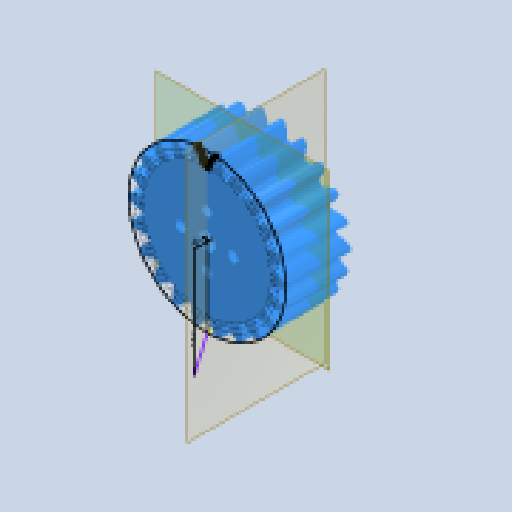
# Autodesk Inventor part: Шестерня
Saved by Autodesk Inventor 2024.2 (Build 282272000, 272)
## iProperties
Created: 2025-11-18
Part Number: Шестерня
Material: Generic
Document SubType Name: Modeling
Designer: katya_notebook
Density: 1 g/cm^3
Appearance: Голубой
Author: katya_notebook
Autodesk Inventor part; units mm, degrees
ref_plane "XZ Plane" through (0, 0, 0) normal (0, 1, 0) x (-1, 0, 0)
ref_plane "XY Plane" through (0, 0, 0) normal (0, 0, 1) x (1, 0, 0)
sketch "Sketch1" plane through (0, 0, 0) normal (0, 0, 1) x (1, 0, 0)
  spline S0 degree 3 poles (-2.783, 24.0561) (-2.7139, 23.9664) (-2.5759, 23.787) (-2.3787, 23.5105) (-2.1892, 23.2287) (-2.0087, 22.941) (-1.838, 22.6474) (-1.6779, 22.3479) (-1.5297, 22.0423) (-1.3949, 21.7305) (-1.2754, 21.4125) (-1.1922, 21.1419) (-1.1368, 20.9223) (-1.1074, 20.7551) (-1.0752, 20.5884) (-1.0286, 20.4249) (-0.9651, 20.2671) (-0.8815, 20.1188) (-0.7929, 20.0079) (-0.7126, 19.9278) (-0.645, 19.8764) (-0.5753, 19.8277) (-0.4987, 19.7907) (-0.4207, 19.7567) (-0.338, 19.7366) (-0.2548, 19.7191) (-0.1414, 19.715) (0, 19.7176) (0.1414, 19.715) (0.2548, 19.7191) (0.338, 19.7366) (0.4207, 19.7567) (0.4987, 19.7907) (0.5753, 19.8277) (0.645, 19.8764) (0.7126, 19.9278) (0.7929, 20.0079) (0.8815, 20.1188) (0.9651, 20.2671) (1.0286, 20.4249) (1.0752, 20.5884) (1.1074, 20.7551) (1.1368, 20.9223) (1.1922, 21.1419) (1.2754, 21.4125) (1.3949, 21.7305) (1.5297, 22.0423) (1.6779, 22.3479) (1.838, 22.6474) (2.0087, 22.941) (2.1892, 23.2287) (2.3787, 23.5105) (2.5759, 23.787) (2.7139, 23.9664) (2.783, 24.0561) knots 0 0 0 0 0.033955 0.067911 0.101866 0.135821 0.169776 0.203731 0.237685 0.271639 0.305591 0.339542 0.356519 0.373494 0.390468 0.407437 0.424408 0.441372 0.458331 0.46682 0.475308 0.483794 0.492283 0.500768 0.509256 0.517742 0.52623 0.543208 0.560186 0.568674 0.57716 0.585647 0.594133 0.602622 0.611107 0.619596 0.628084 0.645044 0.662008 0.678979 0.695948 0.712922 0.729897 0.746874 0.780824 0.814777 0.848731 0.882685 0.916639 0.950594 0.984549 1.018505 1.05246 1.086416 1.086416 1.086416 1.086416
  circle A0 centre (0, 0) radius 19.7166 construction
  circle A1 centre (0, 0) radius 20.6732 construction
  circle A2 centre (0, 0) radius 22 construction
  circle A3 centre (0, 0) radius 24.2166
  point P0 (-2.5775, 23.7858)
  point P1 (-2.38, 23.5096)
  point P2 (-2.1907, 23.2277)
  point P3 (-2.0103, 22.94)
  point P4 (-1.8398, 22.6464)
  point P5 (-1.6799, 22.3468)
  point P6 (-1.5319, 22.0412)
  point P7 (-1.3974, 21.7295)
  point P8 (-1.2787, 21.4114)
  point P9 (-1.1793, 21.0868)
  point P10 (-1.1389, 20.9219)
  point P11 (-1.107, 20.7551)
  point P12 (-1.0728, 20.5889)
  point P13 (-1.0258, 20.4258)
  point P14 (-0.9617, 20.2687)
  point P15 (-0.8777, 20.1213)
  point P16 (-0.7721, 19.9886)
  point P17 (-0.7114, 19.9292)
  point P18 (-0.6446, 19.8768)
  point P19 (-0.5741, 19.8296)
  point P20 (-0.4984, 19.7912)
  point P21 (-0.4199, 19.759)
  point P22 (-0.3379, 19.737)
  point P23 (-0.2545, 19.7215)
  point P24 (-0.1698, 19.7165)
  point P25 (0, 19.7166)
  point P26 (0.1698, 19.7165)
  point P27 (0.2545, 19.7215)
  point P28 (0.3379, 19.737)
  point P29 (0.4199, 19.759)
  point P30 (0.4984, 19.7912)
  point P31 (0.5741, 19.8296)
  point P32 (0.6446, 19.8768)
  point P33 (0.7114, 19.9292)
  point P34 (0.7721, 19.9886)
  point P35 (0.8777, 20.1213)
  point P36 (0.9617, 20.2687)
  point P37 (1.0258, 20.4258)
  point P38 (1.0728, 20.5889)
  point P39 (1.107, 20.7551)
  point P40 (1.1389, 20.9219)
  point P41 (1.1793, 21.0868)
  point P42 (1.2787, 21.4114)
  point P43 (1.3974, 21.7295)
  point P44 (1.5319, 22.0412)
  point P45 (1.6799, 22.3468)
  point P46 (1.8398, 22.6464)
  point P47 (2.0103, 22.94)
  point P48 (2.1907, 23.2277)
  point P49 (2.38, 23.5096)
  point P50 (2.5775, 23.7858)
  constraints: 4 centre point, 2 point on circle, 111 other
extrude "Выдавливание1" add sketch "Sketch1" against normal blind 20
extrude "Выдавливание2" cut sketch "Sketch1" against normal up to surface (20 mm away) contours A3 S0 picked at (-0.4585, 22.7755)
pattern_circular "Круговой массив1" count 22 over 360 about axis through (0, 0, 0) along (0, 0, -1) of "Выдавливание2"
sketch "Эскиз2" plane through (0, 0, 0) normal (1, 0, 0) x (0, 1, 0)
  line L0 (-24.0561, 0) -> (-24.0561, -20) projected
  line L1 (-23.0561, 4) -> (-25.0561, 4)
  line L2 (0, 0) -> (0, -34.2011)
  line L3 (-24.0561, 0) -> (0, 0)
  line L4 (-23.0561, 4) -> (0, 4)
  line L5 (0, 4) -> (0, 0)
  line L6 (-25.0561, 4) -> (-33.7451, 4)
  line L7 (-33.7451, 4) -> (-24.0561, 0)
  dimension "d11" = 2
  dimension "d16" = 4
  constraints: 14 end point, 3 horizontal, 2 parallel, 1 perpendicular, 1 vertical
  measures "d11" distance of L1.start L1.end
  measures "d16" distance of L4.end L2.start
sketch "Эскиз3" plane through (0, 0, 0) normal (0, 0, 1) x (1, 0, 0)
  line L0 (0, 0) -> (0, -47.0266)
  constraints: 2 end point, 1 vertical
ref_plane "РабПлоскость2" through (0, 0, -11) normal (0, 0, -1) x (-1, 0, 0)
sketch "Эскиз5" plane through (0, 0, 0) normal (0, 0, 1) x (1, 0, 0)
  circle A0 centre (0, 0) radius 2.6
  dimension "d18" = 5.2
  constraints: 1 centre point, 1 coincident
  measures "d18" diameter of A0
extrude "Выдавливание4" cut sketch "Эскиз5" against normal blind 18
sketch "Эскиз6" plane through (0, 0, 0) normal (0, 0, 1) x (1, 0, 0)
  circle A0 centre (0, 8) radius 1.5 projected
  circle A1 centre (-8, 0) radius 1.5 projected
  circle A2 centre (0, -8) radius 1.5 projected
  circle A3 centre (8, 0) radius 1.5 projected
  circle A4 centre (-8, 0) radius 1.5
  circle A5 centre (0, 8) radius 1.5
  circle A6 centre (8, 0) radius 1.5
  circle A7 centre (0, -8) radius 1.5
  point P0 (0, 0)
  constraints: 4 centre point, 4 coincident, 4 concentric
extrude "Выдавливание5" cut sketch "Эскиз6" against normal blind 18
equation "\"Модуль\" = 2"
equation "\"Угол_зацепления\" = 20deg"
equation "\"Зазор_профиля_зуба\" = 0.25"
equation "\"Радиус_закругления_зуба\" = 0.35"
equation "\"Диаметр_головки\" = 48.43312"
equation "\"Диаметр_впадин\" = 39.43312"
equation "\"Основной_диаметр\" = 41.34648"
equation "\"Средний_диаметр\" = 44"
equation "\"Ширина_грани\" = 17"
equation "\"Коэффициент_смещения\" = 0.10828"
equation "\"Изменение_высоты_головки_зуба\" = 0"
equation "\"Окружной_шаг\" = 6.283185"
equation "\"Общий_сдвиг_инструмента\" = 0.21656"
equation "\"Внутренний\" = 0"
